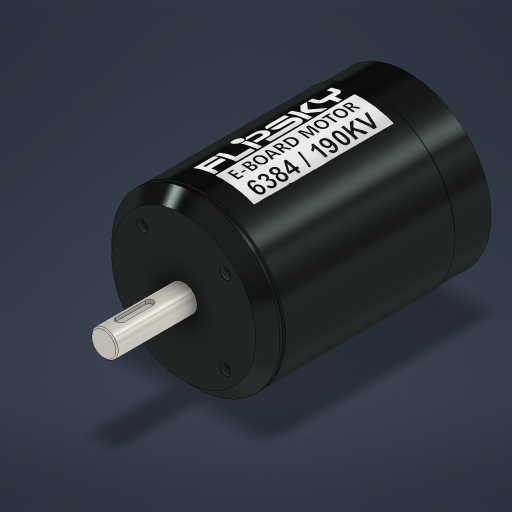
# Autodesk Inventor part: Flipsky E-Board Motor 6384 190KV
Saved by Autodesk Inventor 2024 (Build 280153000, 153)
## iProperties
Created: 2024-04-20
Part Number: Flipsky E-Board Motor 6384 190KV
Material: Generic
Document SubType Name: Modeling
Designer: avsar
Density: 1 g/cm^3
Appearance: Gunmetal - Polished
Author: avsar
Autodesk Inventor part; units mm, degrees
ref_plane "YZ Plane" through (0, 0, 0) normal (1, 0, 0) x (0, 1, 0)
ref_plane "XY Plane" through (0, 0, 0) normal (0, 0, 1) x (1, 0, 0)
sketch "Sketch1" plane through (0, 0, 0) normal (1, 0, 0) x (0, 1, 0)
  line L0 (27, 0) -> (0, 0)
  line L1 (27, 0) -> (31.5, -4.5)
  line L2 (31.5, -4.5) -> (31.5, -5.5)
  line L3 (27, 0) -> (27, -13.1503) construction
  line L4 (31.5, -5.5) -> (30.5, -5.5)
  line L5 (30.5, -5.5) -> (30.5, -6.5)
  line L6 (30.5, -6.5) -> (31.5, -6.5)
  line L7 (31.5, -6.5) -> (31.5, -84)
  line L8 (31.5, -84) -> (0, -84)
  line L9 (0, -84) -> (0, 0)
  dimension "d0" = 27
  dimension "d1" = 31.5
  dimension "d2" = 45
  dimension "d5" = 1
  dimension "d6" = 1
  dimension "d7" = 1
  dimension "d8" = 1
  dimension "d9" = 84
  constraints: 20 end point, 4 perpendicular, 3 horizontal, 2 vertical, 1 coincident
  measures "d0" distance of L0.start L0.end
  measures "d1" distance from line of point (0, 0) L2
  measures "d2" angle of L3 L1
  measures "d5" distance of L1.end L2.end
  measures "d6" distance of L2.end L4.end
  measures "d7" distance of L4.end L5.end
  measures "d8" distance of L5.end L6.end
  measures "d9" vertical distance of L0.start L7.end
revolve "Revolution1" add sketch "Sketch1" angle 360 about axis through (0, 0, -84) along (0, 0, 1)
sketch "Sketch2" plane through (0, 0, 0) normal (0, 0, 1) x (1, 0, 0)
  circle A0 centre (-15.5563, 15.5563) radius 2
  line L0 (-15.5563, 15.5563) -> (0, 0) construction
  line L1 (0, 0) -> (-12.1027, 0) construction
  circle A1 centre (-15.5563, -15.5563) radius 2
  circle A2 centre (15.5563, -15.5563) radius 2
  circle A3 centre (15.5563, 15.5563) radius 2
  dimension "d11" = 4
  dimension "d12" = 22
  dimension "d13" = 45
  dimension "d16" = 360
  constraints: 4 centre point, 4 end point, 1 horizontal, 9 other
  measures "d11" diameter of A0
  measures "d12" distance of L0.start L0.end
  measures "d13" angle of L0 L1
extrude "Extrusion1" cut sketch "Sketch2" against normal blind 5
thread "Thread1" size "M4x0.7" class "6H" standard "ANSI Metric M Profile" full length
thread "Thread2" size "M4x0.7" class "6H" standard "ANSI Metric M Profile" full length
thread "Thread3" size "M4x0.7" class "6H" standard "ANSI Metric M Profile" full length
thread "Thread4" size "M4x0.7" class "6H" standard "ANSI Metric M Profile" full length
sketch "Sketch3" plane through (0, 0, 0) normal (0, 0, 1) x (1, 0, 0)
  circle A0 centre (0, 0) radius 5
  dimension "d28" = 10
  constraints: 1 centre point, 1 coincident
  measures "d28" diameter of A0
extrude "Extrusion2" add sketch "Sketch3" along normal blind 30
chamfer "Chamfer1" distance 0.5 angle 45 1 edges at (-5, 0, 30)
ref_plane "Work Plane1" through (0, 5, 0) normal (0, 1, 0) x (-1, 0, 0)
sketch "Sketch4" plane through (0, 5, 0) normal (0, 1, 0) x (-1, 0, 0)
  line L0 (0, 13) -> (0, 24) construction
  line L1 (1.5, 13) -> (1.5, 24)
  line L2 (-1.5, 24) -> (-1.5, 13)
  arc A0 (-1.5, 13) -> (1.5, 13) centre (0, 13) ccw
  arc A1 (1.5, 24) -> (-1.5, 24) centre (0, 24) ccw
  line L3 (5, 29.5) -> (-5, 29.5) construction
  point P0 (0, 0)
  point P1 (0, 18.5)
  point P2 (0, 29.5)
  point P3 (0, 25.5)
  dimension "d35" = 11
  dimension "d36" = 3
  dimension "d37" = 4
  constraints: 8 end point, 5 point on circle, 4 tangent, 2 centre point, 2 midpoint, 1 parallel, 1 vertical, 1 vertical alignment
  measures "d35" distance of L0.start L0.end
  measures "d36" diameter of A1
  measures "d37" distance of point (0, 29.5) point (0, 25.5)
extrude "Extrusion3" cut sketch "Sketch4" against normal blind 1.5
ref_plane "Work Plane2" through (0, 36, 0) normal (0, 1, 0) x (-1, 0, 0)
sketch "Sketch5" plane through (0, 36, 0) normal (0, 1, 0) x (-1, 0, 0)
  line L0 (14.1999, -66.6752) -> (-12.4029, -66.6752) construction
  line L1 (-12.4029, -66.6752) -> (-12.4029, -14.1495) construction
  line L2 (-12.4029, -14.1495) -> (14.1999, -14.1495) construction
  line L3 (14.1999, -14.1495) -> (14.1999, -66.6752) construction
  point P0 (0, 0)
  constraints: 2 other
decal "Decal1"
sketch "Sketch6" plane through (0, 0, -84) normal (0, 0, -1) x (-1, 0, 0)
  circle A0 centre (0, 0) radius 31.5 projected
  circle A1 centre (0, 0) radius 31
  dimension "d52" = 0.5
  constraints: 1 centre point
  measures "d52" radial gap between concentric circles of A0 A1
extrude "Extrusion4" cut sketch "Sketch6" against normal blind 14
chamfer "Chamfer2" distance 0.5 angle 45 1 edges at (31, 0, -70)
body "Solid1"
